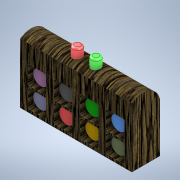
# Autodesk Inventor part: TreasureChestFinalver2
Saved by Autodesk Inventor 2021 (Build 250183000, 183)
## iProperties
Created: 2021-03-02
Part Number: TreasureChestFinalver2
Material: Generic
Document SubType Name: Modeling
Designer: con_c_000
Density: 1 g/cm^3
Appearance: Default
Author: con_c_000
Autodesk Inventor part; units mm, degrees
ref_plane "YZ Plane" through (0, 0, 0) normal (1, 0, 0) x (0, 1, 0)
ref_plane "XZ Plane" through (0, 0, 0) normal (0, 1, 0) x (-1, 0, 0)
ref_plane "XY Plane" through (0, 0, 0) normal (0, 0, 1) x (1, 0, 0)
sketch "Sketch1" plane through (0, 0, 0) normal (0, 1, 0) x (-1, 0, 0)
  line L0 (923.5659, 4.2179) -> (-600.4341, 4.2179)
  line L1 (-600.4341, 4.2179) -> (-600.4341, -300.5821)
  line L2 (-600.4341, -300.5821) -> (923.5659, -300.5821)
  line L3 (923.5659, -300.5821) -> (923.5659, 4.2179)
  point P0 (0, 0)
  dimension "d0" = 1524
  dimension "d1" = 304.8
  constraints: 8 end point, 2 parallel, 1 horizontal, 1 perpendicular
  measures "d0" distance of L2.end L1.end
  measures "d1" distance of L1.end L0.end
extrude "Extrusion1" add sketch "Sketch1" along normal blind 609.6
sketch "Sketch2" plane through (-923.5659, 0, 4.2179) normal (0, 0, 1) x (1, 0, 0)
  circle A0 centre (228.6, 165.1) radius 101.6
  circle A1 centre (584.2, 165.1) radius 101.6
  circle A2 centre (939.8, 165.1) radius 101.6
  circle A3 centre (1295.4, 165.1) radius 101.6
  circle A4 centre (1295.4, 444.5) radius 101.6
  circle A5 centre (939.8, 444.5) radius 101.6
  circle A6 centre (584.2, 444.5) radius 101.6
  circle A7 centre (228.6, 444.5) radius 101.6
  line L0 (1524, 0) -> (1524, 609.6) projected
  line L1 (0, 0) -> (0, 609.6) projected
  line L2 (0, 609.6) -> (1524, 609.6) projected
  point P0 (923.5659, 0)
  dimension "d11" = 203.2
  dimension "d19" = 355.6
  dimension "d20" = 355.6
  dimension "d21" = 165.1
  dimension "d22" = 279.4
  dimension "d23" = 355.6
  dimension "d24" = 228.6
  constraints: 8 centre point, 7 equal radius, 6 horizontal alignment, 4 vertical alignment
  measures "d11" diameter of A7
  measures "d19" distance of A6.centre A5.centre
  measures "d20" distance of A4.centre A5.centre
  measures "d21" distance from line of L2 A7.centre
  measures "d22" distance of A0.centre A7.centre
  measures "d23" distance of A6.centre A7.centre
  measures "d24" distance from line of L1 A7.centre
extrude "Extrusion2" add sketch "Sketch2" along normal blind 25.4
sketch "Sketch3" plane through (-923.5659, 0, 4.2179) normal (0, 0, 1) x (1, 0, 0)
  line L0 (0, 609.6) -> (1524, 609.6) projected
  line L1 (0, 609.6) -> (1524, 609.6)
  line L2 (1524, 609.6) -> (1524, 0)
  line L3 (1524, 0) -> (0, 0)
  line L4 (0, 0) -> (0, 609.6)
  line L5 (101.6, 571.5) -> (355.6, 571.5)
  line L6 (355.6, 571.5) -> (355.6, 317.5)
  line L7 (355.6, 317.5) -> (101.6, 317.5)
  line L8 (101.6, 317.5) -> (101.6, 571.5)
  line L9 (457.2, 317.5) -> (711.2, 317.5)
  line L10 (711.2, 317.5) -> (711.2, 571.5)
  line L11 (711.2, 571.5) -> (457.2, 571.5)
  line L12 (457.2, 571.5) -> (457.2, 317.5)
  line L13 (812.8, 571.5) -> (1066.8, 571.5)
  line L14 (1066.8, 571.5) -> (1066.8, 317.5)
  line L15 (1066.8, 317.5) -> (812.8, 317.5)
  line L16 (812.8, 317.5) -> (812.8, 571.5)
  line L17 (1168.4, 317.5) -> (1422.4, 317.5)
  line L18 (1422.4, 317.5) -> (1422.4, 571.5)
  line L19 (1422.4, 571.5) -> (1168.4, 571.5)
  line L20 (1168.4, 571.5) -> (1168.4, 317.5)
  line L21 (101.6, 292.1) -> (355.6, 292.1)
  line L22 (355.6, 292.1) -> (355.6, 38.1)
  line L23 (355.6, 38.1) -> (101.6, 38.1)
  line L24 (101.6, 38.1) -> (101.6, 292.1)
  line L25 (457.2, 38.1) -> (711.2, 38.1)
  line L26 (711.2, 38.1) -> (711.2, 292.1)
  line L27 (711.2, 292.1) -> (457.2, 292.1)
  line L28 (457.2, 292.1) -> (457.2, 38.1)
  line L29 (812.8, 292.1) -> (1066.8, 292.1)
  line L30 (1066.8, 292.1) -> (1066.8, 38.1)
  line L31 (1066.8, 38.1) -> (812.8, 38.1)
  line L32 (812.8, 38.1) -> (812.8, 292.1)
  line L33 (1168.4, 38.1) -> (1422.4, 38.1)
  line L34 (1422.4, 38.1) -> (1422.4, 292.1)
  line L35 (1422.4, 292.1) -> (1168.4, 292.1)
  line L36 (1168.4, 292.1) -> (1168.4, 38.1)
  line L37 (0, 0) -> (1524, 0) projected
  point P0 (923.5659, 0)
  dimension "d25" = 254
  dimension "d26" = 254
  dimension "d27" = 38.1
  dimension "d28" = 101.6
  dimension "d29" = 101.6
  dimension "d30" = 101.6
  dimension "d31" = 101.6
  dimension "d32" = 0
  dimension "d33" = 0
  dimension "d34" = 0
  dimension "d35" = 254
  dimension "d36" = 25.4
  dimension "d37" = 0
  dimension "d52" = 0
  constraints: 72 end point, 17 parallel, 13 point on line, 10 horizontal, 9 perpendicular, 5 equal length, 1 collinear
  measures "d25" distance of L5.start L5.end
  measures "d26" distance of L7.end L5.start
  measures "d27" distance between parallel lines of L0 L5
  measures "d28" distance between parallel lines of L6 L12
  measures "d29" distance between parallel lines of L4 L8
  measures "d30" distance between parallel lines of L16 L10
  measures "d31" distance between parallel lines of L20 L14
  measures "d32" distance between parallel lines of L13 L19
  measures "d33" distance between parallel lines of L34 L18
  measures "d34" distance between parallel lines of L27 L21
  measures "d35" distance of L23.end L21.start
  measures "d36" distance between parallel lines of L7 L21
  measures "d37" distance between parallel lines of L25 L31
  measures "d52" distance between parallel lines of L24 L8
extrude "Extrusion3" add sketch "Sketch3" along normal blind 76.2
sketch "Sketch5" plane through (0, 609.6, 0) normal (0, 1, 0) x (1, 0, 0)
  line L0 (600.4341, 300.5821) -> (600.4341, -80.4179) projected
  line L1 (600.4341, 300.5821) -> (-923.5659, 300.5821) projected
  line L2 (-923.5659, 300.5821) -> (-923.5659, -80.4179) projected
  line L3 (600.4341, -80.4179) -> (-923.5659, -80.4179) projected
  point P0 (0, 0)
extrude "Extrusion4" add sketch "Sketch5" along normal blind 254
sketch "Sketch6" plane through (-923.5659, 0, -300.5821) normal (-1, 0, 0) x (0, 0, 1)
  line L0 (381, 0) -> (381, 863.6) projected
  line L1 (0, 0) -> (0, 863.6) projected
  arc A0 (381, 815.471) -> (0, 676.7983) centre (235.994, 621.1409) ccw
  line L2 (381, 815.471) -> (0, 676.7983) construction
  line L3 (381, 815.471) -> (786.4517, 815.471) construction
  line L4 (0, 676.7983) -> (381, 676.7983)
  line L5 (381, 676.7983) -> (381, 863.6)
  line L6 (381, 863.6) -> (0, 863.6)
  line L7 (0, 863.6) -> (0, 676.7983)
  point P0 (300.5821, 0)
  point P1 (0, 863.6)
  point P2 (0, 971.0107)
  point P3 (233.8722, 863.6)
  point P4 (238.1158, 863.6)
  dimension "d42" = 160
  constraints: 12 end point, 2 horizontal, 2 parallel, 2 point on circle, 2 point on line, 1 centre point, 1 equal length, 1 perpendicular
  measures "d42" angle of L2 L3
extrude "Extrusion5" cut sketch "Sketch6" against normal through all contours A0 L6 L0 | L1 L6 A0
ref_plane "Work Plane1" through (-923.5659, 863.6093, -64.5881) normal (0, -1, 0) x (1, 0, 0)
sketch "Sketch7" plane through (-923.5659, 863.6093, -64.5881) normal (0, -1, 0) x (1, 0, 0)
  circle A0 centre (635, 0.1041) radius 63.5
  circle A1 centre (889, 0.1041) radius 63.5
  line L0 (1524, -235.994) -> (1524, 145.006) projected
  line L1 (0, 145.006) -> (0, -235.994) projected
  point P0 (923.5659, 64.5881)
  dimension "d45" = 127
  dimension "d46" = 127
  dimension "d47" = 635
  dimension "d48" = 635
  constraints: 2 centre point
  measures "d45" diameter of A0
  measures "d46" diameter of A1
  measures "d47" distance from line of L0 A1.centre
  measures "d48" distance from line of L1 A0.centre
extrude "Extrusion6" add sketch "Sketch7" along normal mid plane 254 from surface at 0
fillet "Fillet1" radius 25.4 2 edges at (-352.0659, 990.6093, -64.4839) (-98.0659, 990.6093, -64.4839)
equation "\"d19\" = d14"
equation "\"d20\" = d14"
equation "\"d23\" = d14"
equation "\"d26\" = d25"
equation "\"d30\" = d28"
equation "\"d31\" = d28"
equation "\"d35\" = d25"
equation "\"d14\" = 355.6"
body "Solid1"
